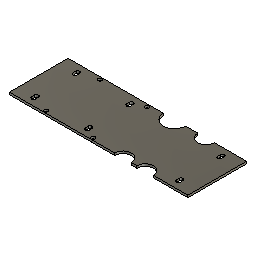
Back MotorController Holder v1 (Autodesk Fusion 360 design; units mm, degrees)
Autodesk Fusion 360 part; units mm, degrees
sketch "Sketch1" plane through (0, 0, 0) normal (0, 0, 1) x (1, 0, 0)
  line L0 (80.5, -26.5) -> (-80.5, -26.5)
  line L1 (-80.5, -26.5) -> (-80.5, 26.5)
  line L2 (-80.5, 26.5) -> (80.5, 26.5)
  line L3 (80.5, 26.5) -> (80.5, -26.5)
  line L4 (80.5, -26.5) -> (-80.5, 26.5) construction
  line L5 (-80.5, -26.5) -> (80.5, 26.5) construction
  dimension "d1" = 161
  dimension "d2" = 53
  constraint horizontal L0
  constraint perpendicular L0 L1
  constraint parallel L0 L2
  constraint parallel L1 L3
  constraint coincident L4 origin
  constraint coincident L5 origin
  measures "d1" distance of L1.end L2.end
  measures "d2" distance of L0.end L1.end
extrude "Extrude1" add sketch "Sketch1" along normal blind 2
sketch "Sketch3" plane through (0, 0, 2) normal (0, 0, 1) x (-1, 0, 0)
  line L0 (-80.5, -26.5) -> (80.5, -26.5)
  line L1 (80.5, -26.5) -> (80.5, 26.5)
  line L2 (80.5, 26.5) -> (-80.5, 26.5)
  line L3 (-80.5, 26.5) -> (-80.5, -26.5)
  circle A0 centre (49.5, -24.1197) radius 1.75
  dimension "d26" = 3.5
  dimension "d72" = 130
  measures "d26" diameter of A0
  measures "d72" distance of L3 A0.centre
extrude "Extrude3" cut sketch "Sketch3" against normal blind 2 contours A0
pattern_linear "R-Pattern4" count 2 spacing 42.5 along (1, 0, 0) count 2 spacing 48.5 along (0, -1, 0) of "Extrude3"
sketch "Sketch6" plane through (0, 0, 2) normal (0, 0, 1) x (-1, 0, 0)
  circle A0 centre (7, 24.3803) radius 1.75
  circle A1 centre (49.5, 24.3803) radius 1.75
  circle A2 centre (7, -24.1197) radius 1.75
  circle A3 centre (49.5, -24.1197) radius 1.75
  line L0 (-80.5, -26.5) -> (80.5, -26.5)
  line L1 (80.5, -26.5) -> (80.5, 26.5)
  line L2 (80.5, 26.5) -> (-80.5, 26.5)
  line L3 (-80.5, 26.5) -> (-80.5, -26.5)
  line L4 (63.4785, -15.65) -> (66.9785, -15.65)
  line L5 (66.9785, -15.65) -> (66.9785, -21.65)
  line L6 (66.9785, -21.65) -> (63.4785, -21.65)
  line L7 (63.4785, -21.65) -> (63.4785, -15.65)
  line L8 (63.4785, -15.65) -> (66.9785, -21.65) construction
  line L9 (66.9785, -15.65) -> (63.4785, -21.65) construction
  point P0 (65.2285, -18.65)
  dimension "d50" = 3.5
  dimension "d51" = 6
  constraint horizontal L4
  constraint perpendicular L4 L5
  constraint parallel L4 L6
  constraint parallel L5 L7
  constraint coincident L8 P0
  constraint coincident L9 P0
  measures "d50" distance of L5.end L6.end
  measures "d51" distance of L4.end L5.end
extrude "Extrude5" cut sketch "Sketch6" against normal blind 2 contours L4 L5 L6 L7
fillet "Fillet1" radius 1.5 4 edges at (-66.9785, 21.65, 1) (-63.4785, 21.65, 1) (-63.4785, 15.65, 1) (-66.9785, 15.65, 1)
pattern_linear "R-Pattern6" count 2 spacing 37.3 along (0, -1, 0) of "Extrude5", "Fillet1"
pattern_linear "R-Pattern8" count 2 spacing 48.5 along (1, 0, 0) of "Extrude5", "Fillet1", "R-Pattern6"
pattern_linear "R-Pattern9" count 2 spacing 130.457 along (1, 0, 0) of "Extrude5", "Fillet1", "R-Pattern6"
sketch "Sketch7" plane through (0, 0, 2) normal (0, 0, 1) x (-1, 0, 0)
  line L0 (-63.4785, 20.15) -> (-63.4785, 17.15)
  arc A0 (-64.9785, 15.65) -> (-63.4785, 17.15) centre (-64.9785, 17.15) ccw
  line L1 (-64.9785, 15.65) -> (-65.4785, 15.65)
  arc A1 (-66.9785, 17.15) -> (-65.4785, 15.65) centre (-65.4785, 17.15) ccw
  line L2 (-66.9785, 17.15) -> (-66.9785, 20.15)
  arc A2 (-65.4785, 21.65) -> (-66.9785, 20.15) centre (-65.4785, 20.15) ccw
  line L3 (-65.4785, 21.65) -> (-64.9785, 21.65)
  arc A3 (-63.4785, 20.15) -> (-64.9785, 21.65) centre (-64.9785, 20.15) ccw
  line L4 (-63.4785, -17.15) -> (-63.4785, -20.15)
  arc A4 (-64.9785, -21.65) -> (-63.4785, -20.15) centre (-64.9785, -20.15) ccw
  line L5 (-64.9785, -21.65) -> (-65.4785, -21.65)
  arc A5 (-66.9785, -20.15) -> (-65.4785, -21.65) centre (-65.4785, -20.15) ccw
  line L6 (-66.9785, -20.15) -> (-66.9785, -17.15)
  arc A6 (-65.4785, -15.65) -> (-66.9785, -17.15) centre (-65.4785, -17.15) ccw
  line L7 (-65.4785, -15.65) -> (-64.9785, -15.65)
  arc A7 (-63.4785, -17.15) -> (-64.9785, -15.65) centre (-64.9785, -17.15) ccw
  line L8 (18.4785, 20.15) -> (18.4785, 17.15)
  arc A8 (16.9785, 15.65) -> (18.4785, 17.15) centre (16.9785, 17.15) ccw
  line L9 (16.9785, 15.65) -> (16.4785, 15.65)
  arc A9 (14.9785, 17.15) -> (16.4785, 15.65) centre (16.4785, 17.15) ccw
  line L10 (14.9785, 17.15) -> (14.9785, 20.15)
  arc A10 (16.4785, 21.65) -> (14.9785, 20.15) centre (16.4785, 20.15) ccw
  line L11 (16.4785, 21.65) -> (16.9785, 21.65)
  arc A11 (18.4785, 20.15) -> (16.9785, 21.65) centre (16.9785, 20.15) ccw
  line L12 (18.4785, -17.15) -> (18.4785, -20.15)
  arc A12 (16.9785, -21.65) -> (18.4785, -20.15) centre (16.9785, -20.15) ccw
  line L13 (16.9785, -21.65) -> (16.4785, -21.65)
  arc A13 (14.9785, -20.15) -> (16.4785, -21.65) centre (16.4785, -20.15) ccw
  line L14 (14.9785, -20.15) -> (14.9785, -17.15)
  arc A14 (16.4785, -15.65) -> (14.9785, -17.15) centre (16.4785, -17.15) ccw
  line L15 (16.4785, -15.65) -> (16.9785, -15.65)
  arc A15 (18.4785, -17.15) -> (16.9785, -15.65) centre (16.9785, -17.15) ccw
  line L16 (66.9785, 20.15) -> (66.9785, 17.15)
  arc A16 (65.4785, 15.65) -> (66.9785, 17.15) centre (65.4785, 17.15) ccw
  line L17 (65.4785, 15.65) -> (64.9785, 15.65)
  arc A17 (63.4785, 17.15) -> (64.9785, 15.65) centre (64.9785, 17.15) ccw
  line L18 (63.4785, 17.15) -> (63.4785, 20.15)
  arc A18 (64.9785, 21.65) -> (63.4785, 20.15) centre (64.9785, 20.15) ccw
  line L19 (64.9785, 21.65) -> (65.4785, 21.65)
  arc A19 (66.9785, 20.15) -> (65.4785, 21.65) centre (65.4785, 20.15) ccw
  line L20 (66.9785, -17.15) -> (66.9785, -20.15)
  arc A20 (65.4785, -21.65) -> (66.9785, -20.15) centre (65.4785, -20.15) ccw
  line L21 (65.4785, -21.65) -> (64.9785, -21.65)
  arc A21 (63.4785, -20.15) -> (64.9785, -21.65) centre (64.9785, -20.15) ccw
  line L22 (63.4785, -20.15) -> (63.4785, -17.15)
  arc A22 (64.9785, -15.65) -> (63.4785, -17.15) centre (64.9785, -17.15) ccw
  line L23 (64.9785, -15.65) -> (65.4785, -15.65)
  arc A23 (66.9785, -17.15) -> (65.4785, -15.65) centre (65.4785, -17.15) ccw
  circle A24 centre (7, 24.3803) radius 1.75
  circle A25 centre (49.5, 24.3803) radius 1.75
  circle A26 centre (7, -24.1197) radius 1.75
  circle A27 centre (49.5, -24.1197) radius 1.75
  line L24 (-80.5, -26.5) -> (80.5, -26.5)
  line L25 (80.5, -26.5) -> (80.5, 26.5)
  line L26 (80.5, 26.5) -> (-80.5, 26.5)
  line L27 (-80.5, 26.5) -> (-80.5, -26.5)
  circle A28 centre (-15.5, -26.5) radius 10
  dimension "d73" = 20
  dimension "d74" = 96
  constraint coincident L24 A28.centre
  measures "d73" diameter of A28
  measures "d74" distance of L25 A28.centre
extrude "Extrude6" cut sketch "Sketch7" against normal blind 2 contours L24 A28 picked at (-16.8366, -22.167)
sketch "Sketch8" plane through (0, 0, 2) normal (0, 0, 1) x (-1, 0, 0)
  arc A0 (-5.5, -26.5) -> (-25.5, -26.5) centre (-15.5, -26.5) ccw
  line L0 (-5.5, -26.5) -> (80.5, -26.5)
  line L1 (80.5, -26.5) -> (80.5, 26.5)
  line L2 (80.5, 26.5) -> (-80.5, 26.5)
  line L3 (-80.5, 26.5) -> (-80.5, -26.5)
  line L4 (-80.5, -26.5) -> (-25.5, -26.5)
  line L5 (-63.4785, 20.15) -> (-63.4785, 17.15)
  arc A1 (-64.9785, 15.65) -> (-63.4785, 17.15) centre (-64.9785, 17.15) ccw
  line L6 (-64.9785, 15.65) -> (-65.4785, 15.65)
  arc A2 (-66.9785, 17.15) -> (-65.4785, 15.65) centre (-65.4785, 17.15) ccw
  line L7 (-66.9785, 17.15) -> (-66.9785, 20.15)
  arc A3 (-65.4785, 21.65) -> (-66.9785, 20.15) centre (-65.4785, 20.15) ccw
  line L8 (-65.4785, 21.65) -> (-64.9785, 21.65)
  arc A4 (-63.4785, 20.15) -> (-64.9785, 21.65) centre (-64.9785, 20.15) ccw
  line L9 (-63.4785, -17.15) -> (-63.4785, -20.15)
  arc A5 (-64.9785, -21.65) -> (-63.4785, -20.15) centre (-64.9785, -20.15) ccw
  line L10 (-64.9785, -21.65) -> (-65.4785, -21.65)
  arc A6 (-66.9785, -20.15) -> (-65.4785, -21.65) centre (-65.4785, -20.15) ccw
  line L11 (-66.9785, -20.15) -> (-66.9785, -17.15)
  arc A7 (-65.4785, -15.65) -> (-66.9785, -17.15) centre (-65.4785, -17.15) ccw
  line L12 (-65.4785, -15.65) -> (-64.9785, -15.65)
  arc A8 (-63.4785, -17.15) -> (-64.9785, -15.65) centre (-64.9785, -17.15) ccw
  line L13 (18.4785, 20.15) -> (18.4785, 17.15)
  arc A9 (16.9785, 15.65) -> (18.4785, 17.15) centre (16.9785, 17.15) ccw
  line L14 (16.9785, 15.65) -> (16.4785, 15.65)
  arc A10 (14.9785, 17.15) -> (16.4785, 15.65) centre (16.4785, 17.15) ccw
  line L15 (14.9785, 17.15) -> (14.9785, 20.15)
  arc A11 (16.4785, 21.65) -> (14.9785, 20.15) centre (16.4785, 20.15) ccw
  line L16 (16.4785, 21.65) -> (16.9785, 21.65)
  arc A12 (18.4785, 20.15) -> (16.9785, 21.65) centre (16.9785, 20.15) ccw
  line L17 (18.4785, -17.15) -> (18.4785, -20.15)
  arc A13 (16.9785, -21.65) -> (18.4785, -20.15) centre (16.9785, -20.15) ccw
  line L18 (16.9785, -21.65) -> (16.4785, -21.65)
  arc A14 (14.9785, -20.15) -> (16.4785, -21.65) centre (16.4785, -20.15) ccw
  line L19 (14.9785, -20.15) -> (14.9785, -17.15)
  arc A15 (16.4785, -15.65) -> (14.9785, -17.15) centre (16.4785, -17.15) ccw
  line L20 (16.4785, -15.65) -> (16.9785, -15.65)
  arc A16 (18.4785, -17.15) -> (16.9785, -15.65) centre (16.9785, -17.15) ccw
  line L21 (66.9785, 20.15) -> (66.9785, 17.15)
  arc A17 (65.4785, 15.65) -> (66.9785, 17.15) centre (65.4785, 17.15) ccw
  line L22 (65.4785, 15.65) -> (64.9785, 15.65)
  arc A18 (63.4785, 17.15) -> (64.9785, 15.65) centre (64.9785, 17.15) ccw
  line L23 (63.4785, 17.15) -> (63.4785, 20.15)
  arc A19 (64.9785, 21.65) -> (63.4785, 20.15) centre (64.9785, 20.15) ccw
  line L24 (64.9785, 21.65) -> (65.4785, 21.65)
  arc A20 (66.9785, 20.15) -> (65.4785, 21.65) centre (65.4785, 20.15) ccw
  line L25 (66.9785, -17.15) -> (66.9785, -20.15)
  arc A21 (65.4785, -21.65) -> (66.9785, -20.15) centre (65.4785, -20.15) ccw
  line L26 (65.4785, -21.65) -> (64.9785, -21.65)
  arc A22 (63.4785, -20.15) -> (64.9785, -21.65) centre (64.9785, -20.15) ccw
  line L27 (63.4785, -20.15) -> (63.4785, -17.15)
  arc A23 (64.9785, -15.65) -> (63.4785, -17.15) centre (64.9785, -17.15) ccw
  line L28 (64.9785, -15.65) -> (65.4785, -15.65)
  arc A24 (66.9785, -17.15) -> (65.4785, -15.65) centre (65.4785, -17.15) ccw
  circle A25 centre (7, 24.3803) radius 1.75
  circle A26 centre (49.5, 24.3803) radius 1.75
  circle A27 centre (7, -24.1197) radius 1.75
  circle A28 centre (49.5, -24.1197) radius 1.75
  circle A29 centre (-41.9978, 26.5) radius 7.5
  dimension "d77" = 15
  constraint coincident L2 A29.centre
  measures "d77" diameter of A29
extrude "Extrude7" cut sketch "Sketch8" against normal blind 2 contours L2 A29 picked at (-42.9111, 24.1728)
sketch "Sketch9" plane through (0, 0, 0) normal (1, 0, 0) x (0, 1, 0)
pattern_linear "R-Pattern10" count 2 spacing 20 along (-1, 0, 0) of "Extrude7"
sketch "Sketch10" plane through (0, 0, 2) normal (0, 0, 1) x (-1, 0, 0)
  arc A0 (-29.4978, 26.5) -> (-14.4978, 26.5) centre (-21.9978, 26.5) ccw
  line L0 (-29.4978, 26.5) -> (-34.4978, 26.5)
  arc A1 (-49.4978, 26.5) -> (-34.4978, 26.5) centre (-41.9978, 26.5) ccw
  line L1 (-49.4978, 26.5) -> (-80.5, 26.5)
  line L2 (-80.5, 26.5) -> (-80.5, -26.5)
  line L3 (-80.5, -26.5) -> (-25.5, -26.5)
  arc A2 (-5.5, -26.5) -> (-25.5, -26.5) centre (-15.5, -26.5) ccw
  line L4 (-5.5, -26.5) -> (80.5, -26.5)
  line L5 (80.5, -26.5) -> (80.5, 26.5)
  line L6 (80.5, 26.5) -> (-14.4978, 26.5)
  line L7 (-63.4785, 20.15) -> (-63.4785, 17.15)
  arc A3 (-64.9785, 15.65) -> (-63.4785, 17.15) centre (-64.9785, 17.15) ccw
  line L8 (-64.9785, 15.65) -> (-65.4785, 15.65)
  arc A4 (-66.9785, 17.15) -> (-65.4785, 15.65) centre (-65.4785, 17.15) ccw
  line L9 (-66.9785, 17.15) -> (-66.9785, 20.15)
  arc A5 (-65.4785, 21.65) -> (-66.9785, 20.15) centre (-65.4785, 20.15) ccw
  line L10 (-65.4785, 21.65) -> (-64.9785, 21.65)
  arc A6 (-63.4785, 20.15) -> (-64.9785, 21.65) centre (-64.9785, 20.15) ccw
  line L11 (-63.4785, -17.15) -> (-63.4785, -20.15)
  arc A7 (-64.9785, -21.65) -> (-63.4785, -20.15) centre (-64.9785, -20.15) ccw
  line L12 (-64.9785, -21.65) -> (-65.4785, -21.65)
  arc A8 (-66.9785, -20.15) -> (-65.4785, -21.65) centre (-65.4785, -20.15) ccw
  line L13 (-66.9785, -20.15) -> (-66.9785, -17.15)
  arc A9 (-65.4785, -15.65) -> (-66.9785, -17.15) centre (-65.4785, -17.15) ccw
  line L14 (-65.4785, -15.65) -> (-64.9785, -15.65)
  arc A10 (-63.4785, -17.15) -> (-64.9785, -15.65) centre (-64.9785, -17.15) ccw
  line L15 (18.4785, 20.15) -> (18.4785, 17.15)
  arc A11 (16.9785, 15.65) -> (18.4785, 17.15) centre (16.9785, 17.15) ccw
  line L16 (16.9785, 15.65) -> (16.4785, 15.65)
  arc A12 (14.9785, 17.15) -> (16.4785, 15.65) centre (16.4785, 17.15) ccw
  line L17 (14.9785, 17.15) -> (14.9785, 20.15)
  arc A13 (16.4785, 21.65) -> (14.9785, 20.15) centre (16.4785, 20.15) ccw
  line L18 (16.4785, 21.65) -> (16.9785, 21.65)
  arc A14 (18.4785, 20.15) -> (16.9785, 21.65) centre (16.9785, 20.15) ccw
  line L19 (18.4785, -17.15) -> (18.4785, -20.15)
  arc A15 (16.9785, -21.65) -> (18.4785, -20.15) centre (16.9785, -20.15) ccw
  line L20 (16.9785, -21.65) -> (16.4785, -21.65)
  arc A16 (14.9785, -20.15) -> (16.4785, -21.65) centre (16.4785, -20.15) ccw
  line L21 (14.9785, -20.15) -> (14.9785, -17.15)
  arc A17 (16.4785, -15.65) -> (14.9785, -17.15) centre (16.4785, -17.15) ccw
  line L22 (16.4785, -15.65) -> (16.9785, -15.65)
  arc A18 (18.4785, -17.15) -> (16.9785, -15.65) centre (16.9785, -17.15) ccw
  line L23 (66.9785, 20.15) -> (66.9785, 17.15)
  arc A19 (65.4785, 15.65) -> (66.9785, 17.15) centre (65.4785, 17.15) ccw
  line L24 (65.4785, 15.65) -> (64.9785, 15.65)
  arc A20 (63.4785, 17.15) -> (64.9785, 15.65) centre (64.9785, 17.15) ccw
  line L25 (63.4785, 17.15) -> (63.4785, 20.15)
  arc A21 (64.9785, 21.65) -> (63.4785, 20.15) centre (64.9785, 20.15) ccw
  line L26 (64.9785, 21.65) -> (65.4785, 21.65)
  arc A22 (66.9785, 20.15) -> (65.4785, 21.65) centre (65.4785, 20.15) ccw
  line L27 (66.9785, -17.15) -> (66.9785, -20.15)
  arc A23 (65.4785, -21.65) -> (66.9785, -20.15) centre (65.4785, -20.15) ccw
  line L28 (65.4785, -21.65) -> (64.9785, -21.65)
  arc A24 (63.4785, -20.15) -> (64.9785, -21.65) centre (64.9785, -20.15) ccw
  line L29 (63.4785, -20.15) -> (63.4785, -17.15)
  arc A25 (64.9785, -15.65) -> (63.4785, -17.15) centre (64.9785, -17.15) ccw
  line L30 (64.9785, -15.65) -> (65.4785, -15.65)
  arc A26 (66.9785, -17.15) -> (65.4785, -15.65) centre (65.4785, -17.15) ccw
  circle A27 centre (7, 24.3803) radius 1.75
  circle A28 centre (49.5, 24.3803) radius 1.75
  circle A29 centre (7, -24.1197) radius 1.75
  circle A30 centre (49.5, -24.1197) radius 1.75
  circle A31 centre (-44.0025, -26.5) radius 7.5
  dimension "d84" = 15
  constraint coincident L3 A31.centre
  measures "d84" diameter of A31
extrude "Extrude8" cut sketch "Sketch10" against normal blind 2 contours L3 A31 | L3 A31
